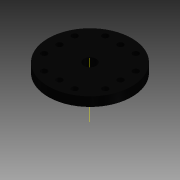
# Autodesk Inventor part: horn01
Saved by Autodesk Inventor 2013 (Build 170138000, 138)
## iProperties
Created: 2013-09-15
Part Number: horn01
Material: ABS Plastic
Document SubType Name: Modeling
Designer: Ian
Density: 1.06 g/cm^3
Mass: 0.950437 g
Surface Area: 10.6704 cm^2
Volume: 0.896639 cm^3
Author: Ian
Autodesk Inventor part; units mm, degrees
ref_plane "YZ Plane" through (0, 0, 0) normal (1, 0, 0) x (0, 1, 0)
ref_plane "XZ Plane" through (0, 0, 0) normal (0, 1, 0) x (-1, 0, 0)
ref_plane "XY Plane" through (0, 0, 0) normal (0, 0, 1) x (1, 0, 0)
sketch "Sketch1" plane through (0, 0, 0) normal (0, 1, 0) x (-1, 0, 0)
  circle A0 centre (0, 0) radius 10.414
  dimension "d0" = 20.828
  constraints: 1 centre point, 1 coincident
  measures "d0" diameter of A0
extrude "Extrusion1" add sketch "Sketch1" along normal blind 2.286
sketch "Sketch2" plane through (0, 0, 0) normal (0, -1, 0) x (1, 0, 0)
  circle A0 centre (0, 0) radius 10.414 projected
  circle A1 centre (0, 0) radius 4.064
  dimension "d3" = 8.128
  constraints: 1 centre point, 1 coincident
  measures "d3" diameter of A1
extrude "Extrusion2" add sketch "Sketch2" along normal blind 4.064 contours A1
sketch "Sketch3" plane through (0, 2.286, 0) normal (0, 1, 0) x (1, 0, 0)
  circle A0 centre (0, 0) radius 10.414 projected
  circle A1 centre (0, 0) radius 7.62 construction
  line L0 (-7.62, 0) -> (-7.62, -7.62) construction
  line L1 (-7.62, -7.62) -> (7.62, -7.62) construction
  line L2 (7.62, -7.62) -> (7.62, 7.62) construction
  line L3 (7.62, 7.62) -> (-7.62, 7.62) construction
  line L4 (-7.62, 7.62) -> (-7.62, 0) construction
  point P0 (0, 7.62)
  point P1 (3.81, 7.62)
  point P2 (-3.81, 7.62)
  point P3 (7.62, 0)
  point P4 (7.62, 3.81)
  point P5 (7.62, -3.81)
  point P6 (-7.62, 3.81)
  point P7 (-7.62, -3.81)
  point P8 (0, -7.62)
  point P9 (-3.81, -7.62)
  point P10 (3.81, -7.62)
  dimension "d6" = 15.24
  dimension "d8" = 7.62
  dimension "d9" = 7.62
  dimension "d10" = 7.62
  dimension "d11" = 3.81
  dimension "d12" = 3.81
  dimension "d13" = 3.81
  dimension "d14" = 3.81
  dimension "d15" = 3.81
  dimension "d16" = 3.81
  dimension "d17" = 3.81
  dimension "d18" = 3.81
  constraints: 10 end point, 6 point on line, 5 midpoint, 3 vertical, 2 coincident, 2 parallel, 1 collinear, 1 horizontal alignment, 1 perpendicular, 2 other
  measures "d8" distance from line of L2 A0.centre
  measures "d9" distance from line of L3 A0.centre
  measures "d10" distance from line of L1 A0.centre
  measures "d11" distance of point (3.81, -7.62) point (0, -7.62)
  measures "d12" distance of point (-3.81, -7.62) point (0, -7.62)
  measures "d13" distance of point (0, 7.62) point (-3.81, 7.62)
  measures "d14" distance of point (3.81, 7.62) point (0, 7.62)
  measures "d15" distance of point (7.62, 3.81) point (7.62, 0)
  measures "d16" distance of point (7.62, -3.81) point (7.62, 0)
  measures "d17" distance of point (-7.62, 3.81) L0.start
  measures "d18" distance of point (-7.62, -3.81) L0.start
hole "Hole1" at (0, 2.286, -7.62) at (3.81, 2.286, -7.62) at (-3.81, 2.286, -7.62) at (7.62, 2.286, 0) at (7.62, 2.286, -3.81) at (7.62, 2.286, 3.81) at (-7.62, 2.286, 0) at (-7.62, 2.286, -3.81) at (-7.62, 2.286, 3.81) at (0, 2.286, 7.62) at (-3.81, 2.286, 7.62) at (3.81, 2.286, 7.62) direction (0, -1, 0) diameter 1.4732 end through all
hole "Hole2" at (0, 2.286, 0) direction (0, -1, 0) diameter 3.048 end through all
body "Solid1"
